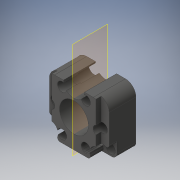
# Autodesk Inventor part: EncoderMount
Saved by Autodesk Inventor 2016 (Build 200138000, 138)
## iProperties
Created: 2016-11-06
Part Number: EncoderMount
Material: Generic
Document SubType Name: Modeling
Designer: brent
Density: 1 g/cm^3
Appearance: Default
Author: brent
Autodesk Inventor part; units mm, degrees
ref_plane "YZ Plane" through (0, 0, 0) normal (1, 0, 0) x (0, 1, 0)
ref_plane "Work Plane1" through (22.7, -20.5, 0) normal (0, 0, 1) x (-1, 0, 0)
sketch "Sketch1" plane through (22.7, -20.5, 0) normal (0, 0, 1) x (-1, 0, 0)
  arc A0 (13.35, 0.5) -> (11.35, -1.5) centre (13.35, -1.5) ccw projected
  line L0 (11.35, -32.85) -> (11.35, -1.5) projected
  arc A1 (15.3515, -24.2) -> (11.35, -32.85) centre (22.7, -32.85) ccw construction
  line L1 (15.3515, -24.2) -> (20.35, -24.2) construction
  line L2 (20.35, -24.2) -> (20.35, -21.2) projected
  arc A2 (25.05, -21.2) -> (20.35, -21.2) centre (22.7, -21.2) ccw projected
  line L3 (25.05, -21.2) -> (25.05, -24.2) projected
  line L4 (25.05, -24.2) -> (30.0485, -24.2) construction
  arc A3 (34.05, -32.85) -> (30.0485, -24.2) centre (22.7, -32.85) ccw construction
  line L5 (34.05, -1.5) -> (34.05, -32.85) projected
  arc A4 (34.05, -1.5) -> (32.05, 0.5) centre (32.05, -1.5) ccw projected
  line L6 (13.35, 0.5) -> (32.05, 0.5) projected
  circle A5 centre (31.7, -1.85) radius 1.25 projected
  circle A6 centre (13.7, -1.85) radius 1.25 projected
  circle A7 centre (22.7, -10.25) radius 4.75 projected
  circle A8 centre (22.7, -10.25) radius 5.5
  arc A9 (18.7, -20.5) -> (26.7, -20.5) centre (22.7, -20.5) ccw construction
  line L7 (26.7, -20.5) -> (18.7, -20.5) construction
  line L8 (18.7, -20.5) -> (26.7, -20.5) construction
  line L9 (26.7, -20.5) -> (34.05, -20.5)
  line L10 (18.7, -20.5) -> (11.35, -20.5)
  arc A10 (26.7, -20.5) -> (18.7, -20.5) centre (22.7, -20.5) ccw
  dimension "d0" = 11
  dimension "d1" = 8
  constraints: 8 end point, 4 point on circle, 3 centre point, 2 coincident, 2 horizontal, 2 midpoint, 2 perpendicular, 2 point on line
  measures "d0" diameter of A8
  measures "d1" diameter of A9
ref_plane "Work Plane2" through (-16.51, -21.68, 12.2) normal (0, 0, -1) x (0, 1, 0)
extrude "Extrusion1" add sketch "Sketch1" along normal up to surface (12.2 mm away) contours L6 A4 L5 L9 A10 L10 L0 A0
fillet "Fillet1" radius 4 2 edges at (11.35, 0, 6.1) (-11.35, 0, 6.1)
sketch "Sketch2" plane through (-9.35, -21, 12.2) normal (0, 0, 1) x (1, 0, 0)
  circle A0 centre (18.35, 2.35) radius 1.25 projected
  circle A1 centre (0.35, 2.35) radius 1.25 projected
  circle A2 centre (0.35, 2.35) radius 3
  circle A3 centre (18.35, 2.35) radius 3
  point P0 (9.35, 21)
  dimension "d5" = 6
  dimension "d6" = 6
  constraints: 2 centre point, 2 coincident
  measures "d5" diameter of A2
  measures "d6" diameter of A3
extrude "Extrusion2" cut sketch "Sketch2" against normal blind 5
sketch "Sketch3" plane through (0, 0, 12.2) normal (0, 0, 1) x (1, 0, 0)
  circle A0 centre (-4.5085, -2.4411) radius 1.65 construction
  circle A1 centre (-4.5085, -18.059) radius 1.65 construction
  circle A2 centre (9.017, -10.25) radius 1.65 construction
  circle A3 centre (9.017, -10.25) radius 1.75
  circle A4 centre (-4.5085, -18.059) radius 1.75
  circle A5 centre (-4.5085, -2.4411) radius 1.75
  point P0 (0, 0)
  dimension "d9" = 3.5
  dimension "d10" = 3.5
  dimension "d11" = 3.5
  constraints: 3 centre point, 3 coincident
  measures "d9" diameter of A3
  measures "d10" diameter of A4
  measures "d11" diameter of A5
extrude "Extrusion3" cut sketch "Sketch3" against normal through all
sketch "Sketch4" plane through (22.7, -20.5, 0) normal (0, 0, -1) x (1, 0, 0)
  circle A0 centre (-27.2085, -2.441) radius 1.75 construction
  circle A1 centre (-13.683, -10.25) radius 1.75 construction
  arc A2 (-25.5069, -17.6502) -> (-26.6207, -19.7073) centre (-27.2085, -18.0589) ccw construction
  circle A3 centre (-22.7, -10.25) radius 5.5 construction
  circle A4 centre (-13.7, -1.85) radius 1.25 construction
  circle A5 centre (-31.7, -1.85) radius 1.25 construction
  line L0 (-11.35, -16.5) -> (-11.35, -1.5) construction
  arc A6 (-13.35, 0.5) -> (-11.35, -1.5) centre (-13.35, -1.5) ccw construction
  line L1 (-13.35, 0.5) -> (-32.05, 0.5) construction
  arc A7 (-34.05, -1.5) -> (-32.05, 0.5) centre (-32.05, -1.5) ccw construction
  line L2 (-34.05, -1.5) -> (-34.05, -16.5) construction
  circle A8 centre (-27.2085, -2.441) radius 2.05
  circle A9 centre (-13.683, -10.25) radius 2.05
  circle A10 centre (-27.2085, -18.0589) radius 2.05
  arc A11 (-18.7, -20.5) -> (-25.5069, -17.6502) centre (-22.7, -20.5) ccw projected
  line L3 (-18.7, -20.5) -> (-15.35, -20.5) projected
  arc A12 (-15.35, -20.5) -> (-11.35, -16.5) centre (-15.35, -16.5) ccw projected
  arc A13 (-34.05, -16.5) -> (-30.05, -20.5) centre (-30.05, -16.5) ccw projected
  line L4 (-30.05, -20.5) -> (-26.7, -20.5) projected
  arc A14 (-26.6207, -19.7073) -> (-26.7, -20.5) centre (-22.7, -20.5) ccw projected
  dimension "d14" = 4.1
  dimension "d15" = 4.1
  dimension "d16" = 4.1
  constraints: 3 centre point, 3 coincident
  measures "d14" diameter of A8
  measures "d15" diameter of A9
  measures "d16" diameter of A10
extrude "Extrusion4" cut sketch "Sketch4" against normal blind 7
fillet "Fillet2" radius 1 4 edges at (11.35, -16.7852, 9.7) (7.1352, -21, 9.7) (-7.1352, -21, 9.7) (-11.35, -16.7852, 9.7)
chamfer "Chamfer1" distance 0.1 angle 45 6 edges at (-6.5585, -18.059, 0) (6.967, -10.25, 0) (-6.3112, -3.4171, 0) (6.967, -10.25, 7) (-6.5585, -18.059, 7) (-6.3112, -3.4171, 7)
ref_plane "Work Plane4" through (0, -19, 0) normal (1, 0, 0) x (0, 0, -1)
sketch "Sketch5" plane through (4, 0, 12.2) normal (0, 0, 1) x (1, 0, 0)
  line L0 (-35.6575, 29.3751) -> (-12.35, 29.3751)
  line L1 (-12.35, 29.3751) -> (-12.35, -28.609)
  line L2 (-12.35, -28.609) -> (-35.6575, -28.609)
  line L3 (-35.6575, -28.609) -> (-35.6575, 29.3751)
  line L4 (-15.35, -4) -> (-15.35, -14.8847) projected
  point P0 (-15.35, 12.35)
  dimension "d37" = 3
  constraints: 8 end point, 2 parallel, 1 horizontal, 1 perpendicular
  measures "d37" distance between parallel lines of L4 L1
extrude "Extrusion5" cut sketch "Sketch5" against normal blind 2
mirror "Mirror1" about plane through (0, -19, 0) normal (1, 0, 0) of "Extrusion5"
sketch "Sketch6" plane through (-9.35, -21, 7.2) normal (0, 0, 1) x (1, 0, 0)
  circle A0 centre (18.35, 2.35) radius 1.25 projected
  circle A1 centre (0.35, 2.35) radius 1.25 projected
  circle A2 centre (0.35, 2.35) radius 1.75
  circle A3 centre (18.35, 2.35) radius 1.75
  point P0 (9.35, 21)
  dimension "d26" = 3.5
  dimension "d27" = 3.5
  constraints: 2 centre point, 2 coincident
  measures "d26" diameter of A2
  measures "d27" diameter of A3
extrude "Extrusion6" cut sketch "Sketch6" against normal through all
pattern_circular "Circular Pattern2" count 6 over 360 about axis through (0, -10.25, 0) along (0, 0, 1) of "Extrusion3", "Extrusion4"
sketch "Sketch7" plane through (22.7, -20.5, 0) normal (0, 0, -1) x (-1, 0, 0)
  circle A0 centre (31.717, 10.25) radius 2.05 projected
  circle A1 centre (13.683, 10.25) radius 2.15 projected
  circle A2 centre (13.683, 10.25) radius 3.5
  circle A3 centre (31.717, 10.25) radius 3.5
  point P0 (22.7, 20.5)
  dimension "d38" = 7
  dimension "d39" = 7
  constraints: 2 centre point, 2 coincident
  measures "d38" diameter of A2
  measures "d39" diameter of A3
equation "\"d10\" = d9"
equation "\"d11\" = d9"
body "Solid1"
